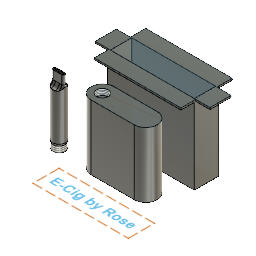
E-Cig v1 (Autodesk Fusion 360 design; units mm, degrees)
Autodesk Fusion 360 part; units mm, degrees
sketch "Sketch1" plane through (0, 0, 0) normal (0, 0, 1) x (1, 0, 0)
  line L0 (-25, -8.2361) -> (25, -8.2361)
  arc A0 (25, -8.2361) -> (25, 18.2361) centre (25, 5) ccw
  line L1 (25, 18.2361) -> (-25, 18.2361)
  arc A1 (-25, 18.2361) -> (-25, -8.2361) centre (-25, 5) ccw
  line L2 (-25, 5) -> (25, 5) construction
  constraint tangent L0 A0
  constraint tangent A0 L1
  constraint parallel L0 L1
  constraint tangent L1 A1
  constraint tangent L0 A1
  constraint horizontal L2
extrude "Extrude1" add sketch "Sketch1" along normal blind 75 makes body 1
sketch "Sketch2" plane through (0, 0, 0) normal (0, 0, -1) x (1, 0, 0)
  arc A0 (-25, 8.2361) -> (-25, -18.2361) centre (-25, -5) ccw
  line L0 (-25, -18.2361) -> (25, -18.2361)
  arc A1 (25, -18.2361) -> (25, 8.2361) centre (25, -5) ccw
  line L1 (25, 8.2361) -> (-25, 8.2361)
  line L2 (-28.0653, -10) -> (-28.0653, 0)
  arc A2 (-28.0653, 0) -> (-31.9347, 0) centre (-30, 0) ccw
  line L3 (-31.9347, 0) -> (-31.9347, -10)
  arc A3 (-31.9347, -10) -> (-28.0653, -10) centre (-30, -10) ccw
  line L4 (-30, -10) -> (-30, 0) construction
  constraint tangent L2 A2
  constraint tangent A2 L3
  constraint parallel L2 L3
  constraint tangent L3 A3
  constraint tangent L2 A3
  constraint perpendicular L0 L4
extrude "Extrude2" cut sketch "Sketch2" against normal blind 10 contours L2 A2 L3 A3 bodies 1
sketch "Sketch3" plane through (0, 0, 0) normal (0, 0, -1) x (1, 0, 0)
  line L0 (-28.0653, 0) -> (-28.0653, -10)
  arc A0 (-31.9347, -10) -> (-28.0653, -10) centre (-30, -10) ccw
  line L1 (-31.9347, -10) -> (-31.9347, 0)
  arc A1 (-28.0653, 0) -> (-31.9347, 0) centre (-30, 0) ccw
  arc A2 (-25, 8.2361) -> (-25, -18.2361) centre (-25, -5) ccw
  line L2 (-25, -18.2361) -> (25, -18.2361)
  arc A3 (25, -18.2361) -> (25, 8.2361) centre (25, -5) ccw
  line L3 (25, 8.2361) -> (-25, 8.2361)
  circle A4 centre (-20, -5) radius 1.7807
extrude "Extrude3" cut sketch "Sketch3" against normal blind 1 contours A4 bodies 1
sketch "Sketch4" plane through (0, 0, 75) normal (0, 0, 1) x (-1, 0, 0)
  arc A0 (25, -18.2361) -> (25, 8.2361) centre (25, -5) ccw
  line L0 (25, 8.2361) -> (-25, 8.2361)
  arc A1 (-25, 8.2361) -> (-25, -18.2361) centre (-25, -5) ccw
  line L1 (-25, -18.2361) -> (25, -18.2361)
  circle A2 centre (25, -5) radius 7.491
  constraint concentric A0 A2
extrude "Extrude4" cut sketch "Sketch4" against normal blind 7 contours A2 bodies 1
thread "Thread1" "ISO Metric profile 15.0 M15x1.5 6H" major diameter 15.2033 minor diameter 13.5262 pitch 1.5 angle 60 resizes the face on face at (-32.4817, 5.3734, 72.6667) on bodies 1
sketch "Sketch5" plane through (0, 0, 75) normal (0, 0, 1) x (-1, 0, 0)
  circle A0 centre (25, -5) radius 6.7631
  arc A1 (25, -18.2361) -> (25, 8.2361) centre (25, -5) ccw
  line L0 (25, 8.2361) -> (-25, 8.2361)
  arc A2 (-25, 8.2361) -> (-25, -18.2361) centre (-25, -5) ccw
  line L1 (-25, -18.2361) -> (25, -18.2361)
sketch "Sketch6" plane through (0, 0, 0) normal (0, 0, 1) x (1, 0, 0)
sketch "Sketch7" plane through (0, 0, 0) normal (0, 0, 1) x (1, 0, 0)
  circle A0 centre (-70, 0) radius 7.3893
extrude "Extrude5" add sketch "Sketch7" along normal blind 55 separate body makes body 2
sketch "Sketch8" plane through (0, 0, 55) normal (0, 0, 1) x (-1, 0, 0)
  circle A0 centre (70, 0) radius 7.3893
  line L0 (75, 2) -> (65, 2)
  arc A1 (65, 2) -> (65, -2) centre (65, 0) ccw
  line L1 (65, -2) -> (75, -2)
  arc A2 (75, -2) -> (75, 2) centre (75, 0) ccw
  line L2 (75, 0) -> (65, 0) construction
  constraint tangent L0 A1
  constraint tangent A1 L1
  constraint parallel L0 L1
  constraint tangent L1 A2
  constraint tangent L0 A2
  constraint horizontal L2
extrude "Extrude6" add sketch "Sketch8" along normal blind 15 contours L0 A1 L1 A2 bodies 2
sketch "Sketch9" plane through (0, 0, 70) normal (0, 0, 1) x (-1, 0, 0)
  arc A0 (75, -2) -> (75, 2) centre (75, 0) ccw
  line L0 (75, 2) -> (65, 2)
  arc A1 (65, 2) -> (65, -2) centre (65, 0) ccw
  line L1 (65, -2) -> (75, -2)
  line L2 (75, 0.7058) -> (65, 0.7058)
  arc A2 (65, 0.7058) -> (65, -0.7058) centre (65, 0) ccw
  line L3 (65, -0.7058) -> (75, -0.7058)
  arc A3 (75, -0.7058) -> (75, 0.7058) centre (75, 0) ccw
  line L4 (75, 0) -> (65, 0) construction
  constraint tangent L2 A2
  constraint tangent A2 L3
  constraint parallel L2 L3
  constraint tangent L3 A3
  constraint tangent L2 A3
  constraint coincident A1.centre A2.centre
  constraint parallel L1 L4
  constraint coincident A0.centre A3.centre
extrude "Extrude7" cut sketch "Sketch9" against normal blind 15 contours L2 A2 L3 A3 bodies 2
fillet "Fillet1" radius 5 4 edges at (-70, 2, 55) (-63, 0, 55) (-70, -2, 55) (-77, 0, 55) on bodies 2
sketch "Sketch10" plane through (0, 0, 0) normal (0, 0, -1) x (1, 0, 0)
  circle A0 centre (-70, 0) radius 7.3893
  circle A1 centre (-70, 0) radius 6.3711
  constraint concentric A0 A1
extrude "Extrude8" add sketch "Sketch10" along normal blind 7 contours A1 bodies 2
thread "Thread2" "ISO Metric profile 14.0 M14x2 6g" major diameter 13.822 minor diameter 11.534 pitch 2 angle 60 resizes the face on face at (-63.6606, 0.6344, -4.6667) on bodies 2
move_body "Move1" bodies 2 to x (1, 0, 0) y (0, 1, 0) z (0, 0, 1) at (0, 0, 7)
fillet "Fillet2" radius 5 1 edges at (-76.8893, -2.6721, 7) on bodies 2
sketch "Sketch11" plane through (0, 0, 0) normal (0, 0, 1) x (1, 0, 0)
  line L0 (50.1124, 35.9139) -> (-50.1124, 35.9139)
  line L1 (-50.1124, 35.9139) -> (-50.1124, 64.0861)
  line L2 (-50.1124, 64.0861) -> (50.1124, 64.0861)
  line L3 (50.1124, 64.0861) -> (50.1124, 35.9139)
  line L4 (50.1124, 35.9139) -> (-50.1124, 64.0861) construction
  line L5 (-50.1124, 35.9139) -> (50.1124, 64.0861) construction
  point P0 (0, 50)
  constraint horizontal L0
  constraint perpendicular L0 L1
  constraint parallel L0 L2
  constraint parallel L1 L3
  constraint coincident L4 P0
  constraint coincident L5 P0
extrude "Extrude9" add sketch "Sketch11" along normal blind 90 separate body makes body 3
sketch "Sketch12" plane through (0, 0, 90) normal (0, 0, 1) x (-1, 0, 0)
  line L0 (-50.1124, -64.0861) -> (50.1124, -64.0861)
  line L1 (50.1124, -64.0861) -> (50.1124, -35.9139)
  line L2 (50.1124, -35.9139) -> (-50.1124, -35.9139)
  line L3 (-50.1124, -35.9139) -> (-50.1124, -64.0861)
  line L4 (48.442, -62.3064) -> (-48.442, -62.3064)
  line L5 (-48.442, -62.3064) -> (-48.442, -37.6936)
  line L6 (-48.442, -37.6936) -> (48.442, -37.6936)
  line L7 (48.442, -37.6936) -> (48.442, -62.3064)
  line L8 (48.442, -62.3064) -> (-48.442, -37.6936) construction
  line L9 (-48.442, -62.3064) -> (48.442, -37.6936) construction
  point P0 (0, -50)
  constraint horizontal L4
  constraint perpendicular L4 L5
  constraint parallel L4 L6
  constraint parallel L5 L7
  constraint coincident L8 P0
  constraint coincident L9 P0
extrude "Extrude10" cut sketch "Sketch12" against normal blind 89 contours L4 L5 L6 L7 bodies 3
sketch "Sketch13" plane through (0, 0, 90) normal (0, 0, 1) x (-1, 0, 0)
  line L0 (-48.442, -62.3064) -> (-48.442, -37.6936)
  line L1 (-48.442, -37.6936) -> (48.442, -37.6936)
  line L2 (48.442, -37.6936) -> (48.442, -62.3064)
  line L3 (48.442, -62.3064) -> (-48.442, -62.3064)
  line L4 (-50.1124, -64.0861) -> (50.1124, -64.0861)
  line L5 (50.1124, -64.0861) -> (50.1124, -35.9139)
  line L6 (50.1124, -35.9139) -> (-50.1124, -35.9139)
  line L7 (-50.1124, -35.9139) -> (-50.1124, -64.0861)
  line L8 (66.1483, -62.3064) -> (34.0764, -62.3064)
  line L9 (34.0764, -62.3064) -> (34.0764, -37.6936)
  line L10 (34.0764, -37.6936) -> (66.1483, -37.6936)
  line L11 (66.1483, -37.6936) -> (66.1483, -62.3064)
  line L12 (66.1483, -62.3064) -> (34.0764, -37.6936) construction
  line L13 (34.0764, -62.3064) -> (66.1483, -37.6936) construction
  line L14 (-66.4824, -62.3064) -> (-33.7423, -62.3064)
  line L15 (-33.7423, -62.3064) -> (-33.7423, -37.6936)
  line L16 (-33.7423, -37.6936) -> (-66.4824, -37.6936)
  line L17 (-66.4824, -37.6936) -> (-66.4824, -62.3064)
  line L18 (-66.4824, -62.3064) -> (-33.7423, -37.6936) construction
  line L19 (-33.7423, -62.3064) -> (-66.4824, -37.6936) construction
  line L20 (50, -80) -> (-50, -80)
  line L21 (-50, -80) -> (-50, -48.1723)
  line L22 (-50, -48.1723) -> (50, -48.1723)
  line L23 (50, -48.1723) -> (50, -80)
  line L24 (50, -80) -> (-50, -48.1723) construction
  line L25 (-50, -80) -> (50, -48.1723) construction
  line L26 (50.1124, -20.5461) -> (-50.1124, -20.5461)
  line L27 (-50.1124, -20.5461) -> (-50.1124, -51.2817)
  line L28 (-50.1124, -51.2817) -> (50.1124, -51.2817)
  line L29 (50.1124, -51.2817) -> (50.1124, -20.5461)
  line L30 (50.1124, -20.5461) -> (-50.1124, -51.2817) construction
  line L31 (-50.1124, -20.5461) -> (50.1124, -51.2817) construction
  point P0 (50.1124, -50)
  point P1 (-50.1124, -50)
  point P2 (0, -64.0861)
  point P3 (0, -35.9139)
  constraint horizontal L8
  constraint perpendicular L8 L9
  constraint parallel L8 L10
  constraint parallel L9 L11
  constraint coincident L12 P0
  constraint coincident L13 P0
  constraint midpoint L5 P0
  constraint horizontal L14
  constraint perpendicular L14 L15
  constraint parallel L14 L16
  constraint parallel L15 L17
  constraint coincident L18 P1
  constraint coincident L19 P1
  constraint midpoint L7 P1
  constraint horizontal L20
  constraint perpendicular L20 L21
  constraint parallel L20 L22
  constraint parallel L21 L23
  constraint coincident L24 P2
  constraint coincident L25 P2
  constraint midpoint L4 P2
  constraint horizontal L26
  constraint perpendicular L26 L27
  constraint parallel L26 L28
  constraint parallel L27 L29
  constraint coincident L30 P3
  constraint coincident L31 P3
  constraint midpoint L6 P3
extrude "Extrude11" add sketch "Sketch13" against normal blind 2 contours L7 L14 L16 L17 L27 | L4 L20 L21 L23 | L6 L26 L27 L29 | L5 L8 L10 L11 L29 bodies 3
sketch "Sketch14" plane through (0, 62.3064, 0) normal (0, -1, 0) x (1, 0, 0)
  line L0 (48.442, 90) -> (-48.442, 90)
  line L1 (-48.442, 90) -> (-48.442, 1)
  line L2 (-48.442, 1) -> (48.442, 1)
  line L3 (48.442, 1) -> (48.442, 90)
sketch "Sketch15" plane through (0, 0, 90) normal (0, 0, 1) x (-1, 0, 0)
  line L0 (-48.442, -62.3064) -> (-48.442, -37.6936)
  line L1 (-48.442, -37.6936) -> (48.442, -37.6936)
  line L2 (48.442, -37.6936) -> (48.442, -62.3064)
  line L3 (48.442, -62.3064) -> (-48.442, -62.3064)
  line L4 (-50.1124, -64.0861) -> (-50, -64.0861)
  line L5 (-50, -64.0861) -> (-50, -80)
  line L6 (-50, -80) -> (50, -80)
  line L7 (50, -80) -> (50, -64.0861)
  line L8 (50, -64.0861) -> (50.1124, -64.0861)
  line L9 (50.1124, -64.0861) -> (50.1124, -62.3064)
  line L10 (50.1124, -62.3064) -> (66.1483, -62.3064)
  line L11 (66.1483, -62.3064) -> (66.1483, -37.6936)
  line L12 (66.1483, -37.6936) -> (50.1124, -37.6936)
  line L13 (50.1124, -37.6936) -> (50.1124, -20.5461)
  line L14 (50.1124, -20.5461) -> (-50.1124, -20.5461)
  line L15 (-50.1124, -20.5461) -> (-50.1124, -37.6936)
  line L16 (-50.1124, -37.6936) -> (-66.4824, -37.6936)
  line L17 (-66.4824, -37.6936) -> (-66.4824, -62.3064)
  line L18 (-66.4824, -62.3064) -> (-50.1124, -62.3064)
  line L19 (-50.1124, -62.3064) -> (-50.1124, -64.0861)
sketch "Sketch16" plane through (0, 0, 0) normal (0, 0, 1) x (1, 0, 0)
  line L0 (-50, -50) -> (60, -50) construction
  line L1 (60, -50) -> (60, -20) construction
  line L2 (60, -20) -> (-50, -20) construction
  line L3 (-50, -20) -> (-50, -50) construction
  dimension "d31" = 10
